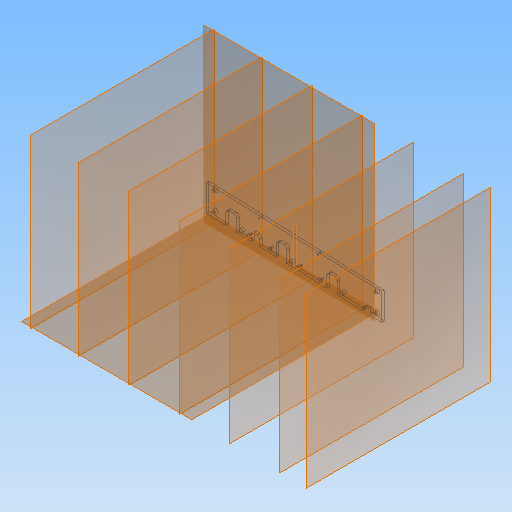
# Autodesk Inventor part: Pancake_Reverse Backboard 2_3 Lanes
Saved by Autodesk Inventor 2018.1 (Build 221171000, 171)
## iProperties
Created: 2019-02-22
Part Number: Pancake_Reverse Backboard 2_3 Lanes
Material: PET Plastic
Document SubType Name: Modeling
Designer: James
Density: 1.541 g/cm^3
Appearance: Polycarbonate - Clear
Author: James
Autodesk Inventor part; units mm, degrees
ref_plane "YZ Plane" through (0, 0, 0) normal (1, 0, 0) x (0, 1, 0)
ref_plane "XZ Plane" through (0, 0, 0) normal (0, 1, 0) x (-1, 0, 0)
ref_plane "XY Plane" through (0, 0, 0) normal (0, 0, 1) x (1, 0, 0)
derived "Pancake_Skeleton.ipt"
ref_plane "Ground" through (0, 0, 0) normal (0, 1, 0) x (-1, 0, 0)
ref_plane "Back" through (0, 0, 0) normal (0, 0, 1) x (1, 0, 0)
ref_plane "LHS" through (0, 0, 0) normal (1, 0, 0) x (0, 1, 0)
ref_plane "Lane 1" through (90, 0, 0) normal (1, 0, 0) x (0, 1, 0)
ref_plane "Lane 2" through (185, 0, 0) normal (1, 0, 0) x (0, 1, 0)
ref_plane "Lane 3" through (280, 0, 0) normal (1, 0, 0) x (0, 1, 0)
ref_plane "Lane 4" through (375, 0, 0) normal (1, 0, 0) x (0, 1, 0)
ref_plane "Lane 5" through (470, 0, 0) normal (1, 0, 0) x (0, 1, 0)
ref_plane "RHS" through (520, 0, 0) normal (1, 0, 0) x (0, 1, 0)
sketch "Sketch1" plane through (0, 0, 0) normal (0, 0, 1) x (1, 0, 0)
  line L0 (0, 75.2308) -> (0, -12.5385) projected
  line L1 (0, 12.6923) -> (330, 0)
  line L2 (330, 0) -> (330, 50)
  line L3 (330, 50) -> (0, 62.6923)
  line L4 (0, 62.6923) -> (0, 12.6923)
  line L5 (-66, 0) -> (396, 0) projected
  line L6 (520, 75.2308) -> (520, -12.5385) projected
  dimension "d31" = 50
  dimension "d134" = 2.203
  dimension "d135" = 190
  constraints: 8 end point, 2 parallel, 1 collinear, 1 point on line, 1 vertical
  measures "d31" distance of L1.end L2.end
  measures "d134" angle of L5 L1
  measures "d135" distance between parallel lines of L6 L2
extrude "Extrusion1" add sketch "Sketch1" along normal blind 5 contours L3 L2 L1 L0
sketch "Sketch2" plane through (0, 0, 5) normal (0, 0, 1) x (1, 0, 0)
  line L0 (90, 75.2308) -> (90, -12.5385) projected
  line L1 (330, 50) -> (0, 62.6923) projected
  line L2 (-85, 0) -> (510, 0) projected
  line L3 (185, 79.6154) -> (185, -13.2692) projected
  line L4 (0, 79.6154) -> (0, -13.2692) projected
  line L5 (0, 12.6923) -> (330, 0) projected
  point P0 (0, 0)
  point P1 (50, 50.7692)
  point P2 (50, 20.7692)
  dimension "d4" = 30
  dimension "d29" = 95
  dimension "d30" = 50
  dimension "d33" = 9.9926
  dimension "d34" = 9.9926
  constraints: 1 vertical alignment
  measures "d4" distance of point (50, 20.769) point (50, 50.769)
  measures "d29" distance between parallel lines of L3 L0
  measures "d30" distance from line of point (50, 50.769) L4
  measures "d33" distance from line of L1 point (50, 50.769)
  measures "d34" distance from line of L5 point (50, 20.769)
hole "Hole1" [suppressed]
pattern_linear "Rectangular Pattern1" [suppressed]
sketch "Sketch3" plane through (0, 0, 0) normal (0, 0, 1) x (1, 0, 0)
  line L0 (330, 50) -> (0, 62.6923) projected
  line L1 (-85, 0) -> (510, 0) projected
  line L2 (0, 79.6154) -> (0, -13.2692) projected
  line L3 (0, 12.6923) -> (330, 0) projected
  line L4 (520, 79.6154) -> (520, -13.2692) projected
  line L5 (330, 0) -> (330, 50) projected
  point P0 (0, 0)
  point P1 (12.5, 55.1923)
  point P2 (12.5, 20.1923)
  point P3 (317.5, 42.5)
  point P4 (317.5, 7.5)
  dimension "d20" = 12.5
  dimension "d36" = 35
  dimension "d39" = 35
  dimension "d41" = 7.5
  dimension "d42" = 7.5
  dimension "d137" = 12.5
  constraints: 2 vertical alignment, 1 other
  measures "d20" distance from line of L2 point (12.5, 55.192)
  measures "d36" distance of point (12.5, 20.192) point (12.5, 55.192)
  measures "d39" distance of point (317.5, 7.5) point (317.5, 42.5)
  measures "d41" vertical distance of L0.start point (317.5, 42.5)
  measures "d42" vertical distance of point (12.5, 55.192) L0.end
  measures "d137" distance from line of L5 point (317.5, 42.5)
hole "Hole2" at (12.5, 55.1923, 0) at (12.5, 20.1923, 0) at (317.5, 42.5, 0) at (317.5, 7.5, 0) direction (0, 0, 1) diameter 4.5 end through all countersink diameter 9.4 countersink angle 90 clearance for "Flat Head Machine Screw" size "M4" standard "Ansi Metric M Profile"
ref_plane "Work Plane10" through (165, 12.6923, 0) normal (-1, 0, 0) x (0, 0, 1)
sketch "Sketch4" plane through (0, 0, 5) normal (0, 0, 1) x (1, 0, 0)
  line L0 (80, 52.1098) -> (78.6548, 17.1357)
  line L1 (479.7045, 36.7366) -> (478.3593, 1.7624)
  line L2 (330, 50) -> (0, 62.6923) projected
  line L3 (0, 12.6923) -> (330, 0) projected
  line L4 (0, 79.6154) -> (0, -13.2692) projected
  line L5 (520, 79.6154) -> (520, -13.2692) projected
  point P0 (0, 0)
  dimension "d43" = 7.5
  dimension "d44" = 7.5
  dimension "d48" = 35
  dimension "d49" = 80
  dimension "d58" = 35
  dimension "d60" = 400
  constraints: 4 end point, 2 perpendicular, 1 other
  measures "d43" distance from line of L2 L0.start
  measures "d44" distance from line of L2 L1.start
  measures "d48" distance of L0.start L0.end
  measures "d49" distance from line of L0.start L4
  measures "d58" distance of L1.start L1.end
  measures "d60" distance of L1.start L0.start
hole "Hole3" [suppressed]
sketch "Sketch5" plane through (0, 0, 5) normal (0, 0, 1) x (1, 0, 0)
  line L0 (0, 75.2308) -> (0, -12.5385) projected
  line L1 (520, 75.2308) -> (520, -12.5385) projected
  line L2 (330, 50) -> (0, 62.6923) projected
  line L3 (330, 0) -> (330, 50) projected
  point P0 (0, 0)
  point P1 (100, 54.8432)
  point P2 (209.9187, 50.6156)
  dimension "d61" = 110
  dimension "d62" = 100
  dimension "d64" = 4
  dimension "d65" = 4
  dimension "d136" = 120.0813
  constraints: 1 other
  measures "d61" distance of point (209.919, 50.616) point (100, 54.843)
  measures "d62" distance from line of L0 point (100, 54.843)
  measures "d64" distance from line of L2 point (209.919, 50.616)
  measures "d65" distance from line of point (100, 54.843) L2
  measures "d136" distance from line of L3 point (209.919, 50.616)
hole "Hole4" at (100, 54.8432, 5) at (209.9187, 50.6156, 5) direction (0, 0, -1) diameter 3.4 end through all clearance for "Flat Head Machine Screw" size "M3" standard "Ansi Metric M Profile"
sketch "Sketch6" plane through (0, 0, 5) normal (0, 0, 1) x (1, 0, 0)
  line L0 (0, 12.6923) -> (330, 0) projected
  line L1 (90, 75.2308) -> (90, -12.5385) projected
  point P0 (0, 0)
  point P1 (65, 16.6971)
  dimension "d74" = 6.5
  dimension "d75" = 25
  measures "d74" distance from line of L0 point (65, 16.697)
  measures "d75" distance from line of L1 point (65, 16.697)
hole "Hole5" at (65, 16.6971, 5) direction (0, 0, -1) diameter 7 end through all
pattern_linear "Rectangular Pattern2" count 3 spacing 95 along (0.9992612, -0.0384331, 0) of "Hole5"
sketch "Sketch7" plane through (0, 0, 5) normal (0, 0, 1) x (1, 0, 0)
  circle A0 centre (65, 16.6971) radius 3.5 projected
  line L0 (-66, 0) -> (396, 0) projected
  line L1 (37, 0) -> (57, 0)
  line L2 (57, 0) -> (57, 38)
  line L3 (57, 38) -> (37, 38)
  line L4 (37, 38) -> (37, 0)
  point P0 (0, 0)
  dimension "d113" = 38
  dimension "d114" = 20
  dimension "d115" = 8
  constraints: 8 end point, 2 parallel, 1 horizontal, 1 perpendicular, 1 point on line
  measures "d113" distance of L3.end L1.start
  measures "d114" distance of L2.end L3.end
  measures "d115" distance from line of A0.centre L2
extrude "Extrusion2" cut sketch "Sketch7" against normal through all contours L4 L3 L2 L0
sketch "Sketch8" plane through (0, 0, 5) normal (0, 0, 1) x (1, 0, 0)
  line L0 (32.5, 65.1923) -> (67.5, 65.1923)
  line L1 (67.5, 65.1923) -> (67.5, 35.1923)
  line L2 (67.5, 35.1923) -> (32.5, 35.1923)
  line L3 (32.5, 35.1923) -> (32.5, 65.1923)
  line L4 (0, 82.6154) -> (0, -13.7692) projected
  circle A0 centre (12.5, 55.1923) radius 2.25 projected
  point P0 (0, 0)
  dimension "d94" = 35
  dimension "d95" = 32.5
  dimension "d96" = 20
  dimension "d97" = 10
  constraints: 8 end point, 2 parallel, 1 horizontal, 1 perpendicular
  measures "d94" distance of L0.start L0.end
  measures "d95" distance between parallel lines of L3 L4
  measures "d96" distance from line of L2 A0.centre
  measures "d97" distance from line of L0 A0.centre
extrude "Extrusion3" [suppressed]
fillet "Fillet1" [suppressed]
pattern_linear "Rectangular Pattern4" [suppressed]
sketch "Sketch9" plane through (0, 0, 5) normal (0, 0, 1) x (1, 0, 0)
  line L0 (100, 0) -> (85, 0)
  line L1 (85, 0) -> (85, 25)
  line L2 (85, 25) -> (100, 25)
  line L3 (100, 25) -> (100, 0)
  line L4 (0, 75.2308) -> (0, -12.5385) projected
  line L5 (-81, 0) -> (486, 0) projected
  line L6 (310, 0) -> (295, 0)
  line L7 (295, 0) -> (295, 10)
  line L8 (295, 10) -> (310, 10)
  line L9 (310, 10) -> (310, 0)
  line L10 (520, 75.2308) -> (520, -12.5385) projected
  line L11 (330, 0) -> (330, 50) projected
  point P0 (0, 0)
  dimension "d104" = 85
  dimension "d105" = 15
  dimension "d106" = 25
  dimension "d107" = 10
  dimension "d108" = 15
  dimension "d138" = 20
  constraints: 16 end point, 4 parallel, 2 horizontal, 2 perpendicular, 1 collinear, 1 point on line
  measures "d104" distance between parallel lines of L1 L4
  measures "d105" distance of L1.end L2.end
  measures "d106" distance of L2.end L0.start
  measures "d107" distance of L8.end L6.start
  measures "d108" distance of L7.end L8.end
  measures "d138" distance between parallel lines of L11 L9
extrude "Extrusion4" cut sketch "Sketch9" against normal through all
fillet "Fillet2" radius 5 4 edges at (85, 25, 2.5) (100, 25, 2.5) (295, 10, 2.5) (310, 10, 2.5)
fillet "Fillet3" radius 5 2 edges at (57, 38, 2.5) (37, 38, 2.5)
pattern_linear "Rectangular Pattern5" count 3 spacing 95 along (0.9992612, -0.0384331, 0) of "Extrusion2", "Fillet3"
sketch "Sketch10" plane through (0, 0, 5) normal (0, 0, 1) x (1, 0, 0)
  line L0 (57, 10.5) -> (85, 9.4231) projected
  line L1 (100, 8.8462) -> (131.9298, 7.6181) projected
  circle A0 centre (65, 16.6971) radius 3.5 projected
  point P0 (0, 0)
  point P1 (80, 16.6206)
  point P2 (119.9704, 15.0832)
  dimension "d120" = 7
  dimension "d121" = 7
  dimension "d122" = 15
  dimension "d123" = 40
  measures "d120" distance from line of point (80, 16.621) L0
  measures "d121" distance from line of L1 point (119.97, 15.083)
  measures "d122" horizontal distance of point (80, 16.621) A0.centre
  measures "d123" distance of point (119.97, 15.083) point (80, 16.621)
hole "Hole6" at (80, 16.6206, 5) at (119.9704, 15.0832, 5) direction (0, 0, -1) diameter 3.4 end through all countersink diameter 6.3 countersink angle 90 clearance for "Flat Head Machine Screw" size "M3" standard "Ansi Metric M Profile"
pattern_linear "Rectangular Pattern6" count 2 spacing 95 along (0.9992612, -0.0384331, 0) of "Hole6"
equation "\"d33\" = d34"
equation "\"d44\" = d43"
equation "\"d58\" = d48"
equation "\"d65\" = d64"
equation "\"d108\" = d105"
equation "\"d121\" = d120"
body "Solid1"
